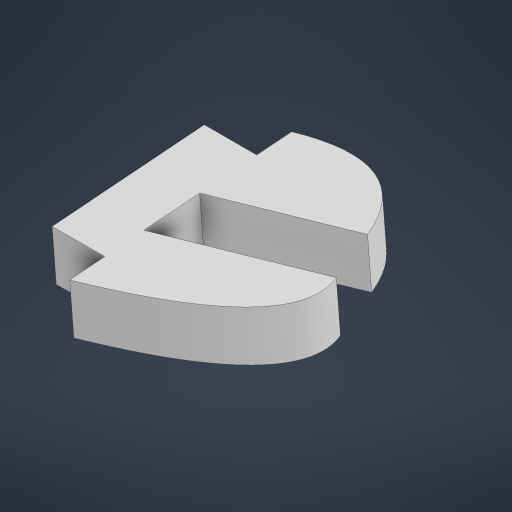
# Autodesk Inventor part: sponson_spanner_bottom_holder
Saved by Autodesk Inventor 2024 (Build 280153000, 153)
## iProperties
Created: 2022-03-22
Part Number: sponson_spanner_bottom_holder
Material: Generic
Document SubType Name: Modeling
Designer: kardo
Density: 1 g/cm^3
Appearance: Default
Mass: 0.292099 g
Surface Area: 4.00251 cm^2
Volume: 0.292099 cm^3
Author: kardo
Autodesk Inventor part; units mm, degrees
ref_plane "YZ Plane" through (0, 0, 0) normal (1, 0, 0) x (0, 1, 0)
ref_plane "XZ Plane" through (0, 0, 0) normal (0, 1, 0) x (-1, 0, 0)
ref_plane "XY Plane" through (0, 0, 0) normal (0, 0, 1) x (1, 0, 0)
derived "parameters_frame.ipt"
derived "stencil_frame.ipt"
sketch "sk_joint_locations" plane through (81.12, 0, 0) normal (1, 0, 0) x (0, 1, 0)
  line L0 (0, 0) -> (122.4, 9.6331) construction
  line L1 (36.465, 28.832) -> (112.2, 28.832) construction
  arc A0 (36.465, 28.832) -> (11.22, 28.376) centre (36.465, -670.197) ccw construction
  line L2 (-241.5001, 19.2432) -> (11.22, 28.376) construction
  line L3 (-345, 16.32) -> (-262.2001, 18.586) construction
  arc A1 (-262.2001, 18.586) -> (-241.5001, 19.2432) centre (-326.8578, 2381.2399) ccw construction
  line L4 (-122.4795, 3121.122) -> (270.8781, -1876.9598) construction
  line L5 (-230.0001, 3089.1136) -> (-230.0001, -1866.0023) construction
  line L6 (-114.9999, 3089.1136) -> (-114.9999, -1866.0023) construction
  line L7 (-345, 3089.1136) -> (-345, -1866.0023) construction
  line L8 (0, 3089.1136) -> (0, -1866.0023) construction
  line L9 (529.622, 47.2379) -> (-602.608, 2.7525) construction
  line L10 (-673.1615, -36.5999) -> (647.9226, 67.3717) construction
  line L11 (189.4528, 29.5173) -> (189.1111, 38.2146) construction
  line L12 (201.105, 36.5853) -> (201.7901, 27.8813) construction
  line L13 (0, 14.144) -> (121.9006, 15.9783) construction
  line L14 (-230.0001, 45.8224) -> (-230.0001, 19.6588) construction
  line L15 (-345, 37.3935) -> (-345, 16.32) construction
  line L16 (-114.9999, 50.9907) -> (-114.9999, 23.8147) construction
  line L17 (0, 52.89) -> (0, 27.9705) construction
  line L18 (119.1768, 50.5875) -> (119.7216, 43.6656) construction
  line L19 (120.2663, 36.7438) -> (119.7216, 43.6656) construction
  line L20 (120.2663, 36.7438) -> (120.8111, 29.822) construction
  line L21 (120.8111, 29.822) -> (121.3559, 22.9001) construction
  line L22 (121.3559, 22.9001) -> (121.9006, 15.9783) construction
  line L23 (0, 14.144) -> (0, 0) construction
  line L24 (112.2, 37.536) -> (112.2, 28.832) construction
  line L25 (112.2, 35.848) -> (112.2, 30.52) construction
  spline S0 degree 4 poles (-345, 37.3935) (-258.8686, 45.1235) (-172.5923, 49.7074) (-86.3167, 52.89) (0, 52.89) knots 0 0 0 0 0 1 1 1 1 1
  spline S1 degree 3 poles (0, 52.89) (92.8353, 52.89) (195.0311, 49.5089) (255, 36.448) knots 0 0 0 0 1 1 1 1
  spline S2 degree 2 poles (122.4, 9.6331) (190.08, 14.9596) (255, 36.448) knots 0 0 0 1 1 1
  point P0 (-122.4795, 3121.122)
  point P1 (270.8781, -1876.9598)
  point P2 (189.282, 33.8659)
  point P3 (201.4475, 32.2333)
  point P4 (134.9575, 11.3411)
  point P5 (-345, 26.8568)
  point P6 (-230.0001, 32.7406)
  point P7 (-114.9999, 37.4027)
  point P8 (0, 40.4303)
  point P9 (112.2, 33.184)
derived "surface_body.ipt"
ref_plane "plane_tunnel_right" through (81.12, 0, 0) normal (1, 0, 0) x (0, 1, 0)
ref_plane "plane_sponson_boittom" through (126.048, 0, 0) normal (0.341579, -0.07374, 0.9369558) x (-0.1718217, 0.9752166, 0.139391)
ref_plane "plane_base" through (81.12, 201.4475, 32.2333) normal (0, -0.9969173, -0.0784591) x (1, 0, 0)
sketch "sk_base" plane through (81.12, 201.4475, 32.2333) normal (0, -0.9969173, -0.0784591) x (1, 0, 0)
  line L0 (0, 3002.8469) -> (0, -1322.6219) projected
  line L1 (-1052.212, 382.4145) -> (452.1952, -164.3452) construction
  line L2 (0, 4.3655) -> (3, 4.3655)
  line L3 (0, -4.3655) -> (3, -4.3655)
  line L4 (3, -4.3655) -> (3, -6.3655)
  line L5 (3, 4.3655) -> (3, 6.3655)
  line L6 (3, 2.1017) -> (11.0736, -0.8326)
  line L7 (3, 0.5057) -> (10.5613, -2.2424) construction
  line L8 (10.0489, -3.6522) -> (3, -1.0903)
  line L9 (3, 2.1017) -> (3, -1.0903)
  line L10 (11.0736, -0.8326) -> (10.0489, -3.6522) construction
  line L11 (11.0736, -0.8326) -> (12.4425, 2.9337) construction
  line L12 (12.4425, 2.9337) -> (3, 6.3655) construction
  spline S0 degree 2 poles (11.0736, -0.8326) (12.4425, 2.9337) (3, 6.3655) knots 1 1 1 2 2 2
  line L13 (10.0489, -3.6522) -> (8.3554, -8.3118) construction
  line L14 (8.3554, -8.3118) -> (3, -6.3655) construction
  spline S1 degree 2 poles (10.0489, -3.6522) (8.3554, -8.3118) (3, -6.3655) knots 1 1 1 2 2 2
  point P0 (-81.12, -16.3286)
  dimension "d10" = 7.5
  dimension "d11" = 3
  dimension "d12" = 3
  dimension "d13" = 2
  dimension "d14" = 2
  constraints: 18 end point, 6 parallel, 4 point on line, 3 collinear, 3 perpendicular, 2 midpoint, 7 other
  measures "d10" distance of L8.start L8.end
  measures "d11" distance of L6.end L8.start
  measures "d12" distance of L2.start L2.end
  measures "d13" distance of L2.end L5.end
  measures "d14" distance of L3.end L4.end
extrude "thicken" add sketch "sk_base" along normal blind 3
equation "\"d10\" = 2.5 * bulkhead_thickness"
equation "\"d11\" = bulkhead_thickness"
equation "\"d12\" = stringer_thickness"
equation "\"d7\" = bulkhead_thickness"
equation "\"bulkhead_thickness\" = 3"
equation "\"stringer_thickness\" = 3"
body "Solid1"
